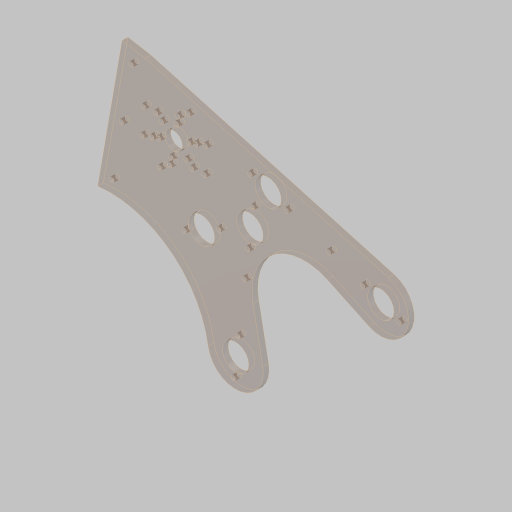
# Autodesk Inventor part: GP7-001
Saved by Autodesk Inventor 2023.5 (Build 275446000, 446)
## iProperties
Created: 2025-02-24
Part Number: GP7-001
Material: Polycarbonate, Smoke
Document SubType Name: Modeling
Designer: dlangdon
Density: 1.2 g/cm^3
Appearance: Polycarbonate - Smoked
Author: dlangdon
Autodesk Inventor part; units mm, degrees
ref_plane "YZ Plane" through (0, 0, 0) normal (1, 0, 0) x (0, 1, 0)
ref_plane "XZ Plane" through (0, 0, 0) normal (0, 1, 0) x (-1, 0, 0)
ref_plane "XY Plane" through (0, 0, 0) normal (0, 0, 1) x (1, 0, 0)
sketch "Sketch1" plane through (0, 0, 0) normal (0, 0, 1) x (1, 0, 0)
  circle A0 centre (78.7027, 64.253) radius 50.8 construction
  circle A1 centre (-78.7027, -64.253) radius 50.8 construction
  circle A2 centre (0, 0) radius 50.8 construction
  line L0 (-39.3513, -32.1265) -> (39.3513, 32.1265) construction
  line L1 (78.7027, 64.253) -> (-78.7027, -64.253) construction
  line L2 (-3.7208, 6.6498) -> (-3.7208, 50.6636) construction
  line L3 (-410.4212, -115.053) -> (454.9708, -115.053) construction
  circle A3 centre (140.9799, -57.903) radius 57.15 construction
  circle A4 centre (78.7027, 64.253) radius 14.2621
  circle A5 centre (-78.7027, -64.253) radius 14.2621
  circle A6 centre (-3.7208, 6.6498) radius 57.15 construction
  circle A7 centre (-78.7027, -64.253) radius 30.1371 construction
  circle A8 centre (78.7027, 64.253) radius 30.1371 construction
  circle A9 centre (-43.5314, 108.1291) radius 14.2621
  line L4 (-43.5314, 108.1291) -> (78.7027, 64.253) construction
  circle A10 centre (78.7027, 64.253) radius 14.2875 construction
  circle A11 centre (-78.7027, -64.253) radius 14.2875 construction
  circle A12 centre (-63.1248, 64.6795) radius 14.2621
  line L5 (-78.7027, -64.253) -> (-63.1248, 64.6795) construction
  circle A13 centre (-63.1248, 64.6795) radius 23.8316 construction
  circle A14 centre (-43.5314, 108.1291) radius 23.8316 construction
  line L6 (20.6869, 58.3256) -> (65.8317, 37.0027)
  line L7 (-49.1354, -58.4201) -> (-59.7901, -4.4114)
  arc A15 (20.6869, 58.3256) -> (-59.7901, -4.4114) centre (-3.7208, 6.6498) ccw
  line L8 (-201.842, 171.7522) -> (-176.8279, 167.3416)
  line L9 (-176.8279, 167.3416) -> (-203.2918, 17.2569) construction
  line L10 (-203.2918, 17.2569) -> (-228.306, 21.6675) construction
  line L11 (-228.306, 21.6675) -> (-201.842, 171.7522) construction
  line L12 (-247.3095, -86.1068) -> (28.2095, -134.6882) construction
  line L13 (-202.9446, 165.4987) -> (190.461, 96.1307) construction
  line L14 (-202.9446, 165.4987) -> (-247.3095, -86.1068) construction
  circle A16 centre (-145.8493, 105.3365) radius 31.75 construction
  line L15 (-65.9834, 41.02) -> (-72.6092, -13.8198) construction
  circle A17 centre (21.9247, 84.6336) radius 9.525 construction
  line L16 (-189.3349, 169.5469) -> (-215.7989, 19.4622) construction
  line L17 (-192.0916, 153.9131) -> (-213.0422, 35.096) construction
  circle A18 centre (-145.8493, 105.3365) radius 17.4625 construction
  circle A19 centre (-145.8493, 105.3365) radius 9.525
  circle A20 centre (-43.5314, 108.1291) radius 30.1816 construction
  line L18 (-201.842, 171.7522) -> (-228.306, 21.6675)
  arc A21 (65.8317, 37.0027) -> (86.8534, 93.267) centre (78.7027, 64.253) ccw
  arc A22 (-108.4816, -68.8852) -> (-49.1354, -58.4201) centre (-78.7027, -64.253) ccw
  line L19 (-145.8493, 105.3365) -> (-129.4399, 111.3091) construction
  line L20 (-111.5388, 117.8245) -> (-180.1598, 92.8485) construction
  circle A23 centre (-180.1598, 92.8485) radius 4.7625 construction
  line L21 (0, 0) -> (-3.7208, 6.6498) construction
  circle A24 centre (78.7027, 64.253) radius 28.6512 construction
  line L22 (66.0948, 38.525) -> (-49.8074, 95.3221) construction
  line L23 (85.335, 92.126) -> (-40.2299, 122.0038) construction
  line L24 (-176.8279, 167.3416) -> (86.8534, 93.267)
  line L25 (-145.8493, 105.3365) -> (-115.7736, 36.5549) construction
  circle A25 centre (-115.7736, 36.5549) radius 31.75 construction
  circle A26 centre (-115.7736, 36.5549) radius 14.2621
  line L26 (-63.1248, 64.6795) -> (-115.7736, 36.5549) construction
  circle A27 centre (-145.8493, 105.3365) radius 25.4 construction
  arc A28 (-108.4816, -68.8852) -> (-228.306, 21.6675) centre (-215.1488, -85.4777) ccw
  circle A29 centre (-145.8493, 105.3365) radius 36.5125 construction
  line L27 (-178.9408, 120.7674) -> (-145.8493, 105.3365) construction
  point P0 (-69.2963, 13.6001)
  point P1 (-202.5669, 94.5046)
  point P2 (-202.5669, 94.5046)
  point P3 (-142.817, 122.5337)
  point P4 (-159.2263, 116.5612)
  point P5 (-162.2587, 99.364)
  point P6 (-148.8816, 88.1393)
  point P7 (-132.4722, 94.1119)
  point P8 (-121.9811, 114.0238)
  point P9 (-141.4386, 130.3506)
  point P10 (-165.3068, 121.6633)
  point P11 (-169.7175, 96.6492)
  point P12 (-150.2599, 80.3224)
  point P13 (-126.3918, 89.0097)
  point P14 (-158.3373, 139.6471)
  point P15 (-180.1598, 92.8485)
  point P16 (-133.3613, 71.026)
  point P17 (-130.4184, 138.4281)
  point P18 (-161.2801, 72.245)
  point P19 (-112.7577, 89.9057)
  dimension "d7" = 101.6
  dimension "d18" = 47.6631
  dimension "d34" = 34.925
  dimension "d65" = 50.8
  dimension "d3" = 50.772
  dimension "d4" = 0
  dimension "d8" = 101.6
  dimension "d9" = 28.5242
  dimension "d10" = 101.6
  dimension "d11" = 114.3
  dimension "d12" = 114.3
  dimension "d13" = 15.875
  dimension "d14" = 15.875
  dimension "d15" = 129.8702
  dimension "d16" = 28.575
  dimension "d17" = 129.8702
  dimension "d19" = 47.6631
  dimension "d22" = 25.4
  dimension "d23" = 152.4
  dimension "d26" = 255.4869
  dimension "d27" = 63.5
  dimension "d30" = 203.2
  dimension "d31" = 10
  dimension "d32" = 19.05
  dimension "d33" = 120.65
  dimension "d35" = 19.05
  dimension "d36" = 6.35
  dimension "d40" = 360
  dimension "d44" = 9.525
  dimension "d55" = 80
  dimension "d56" = 7.62
  dimension "d58" = 57.3024
  dimension "d59" = 63.5
  dimension "d60" = 75.0697
  dimension "d61" = 59.69
  dimension "d62" = 55
  dimension "d68" = 360
  dimension "d70" = 41.275
  dimension "d71" = 60
  dimension "d82" = 360
  dimension "d87" = 360
  dimension "d89" = 45
  dimension "d90" = 6.35
  dimension "d91" = 20.955
  dimension "d92" = 107.95
  constraints: 56 end point, 26 centre point, 24 coincident, 23 point on circle, 14 tangent, 7 midpoint, 6 equal radius, 5 point on line, 4 collinear, 4 parallel, 2 horizontal, 1 concentric, 1 perpendicular, 1 vertical, 39 other
  measures "d3" angle of L2 L0
  measures "d4" distance between parallel lines of L0 L1
  measures "d8" diameter of A2
  measures "d9" diameter of A4
  measures "d10" diameter of A0
  measures "d11" diameter of A3
  measures "d12" diameter of A6
  measures "d13" radial gap between concentric circles of A5 A7
  measures "d14" radial gap between concentric circles of A4 A8
  measures "d15" distance of L4.start L4.end
  measures "d16" diameter of A10
  measures "d17" distance of L5.start L5.end
  measures "d19" diameter of A14
  measures "d22" distance of L9.end L10.end
  measures "d23" distance of L10.end L8.start
  measures "d26" distance of L13.start L12.start
  measures "d27" diameter of A16
  measures "d30" distance from line of point (0, 0) L9
  measures "d31" angle of L3 L12
  measures "d32" diameter of A17
  measures "d33" distance of L17.start L17.end
  measures "d35" diameter of A19
  measures "d36" radial gap between concentric circles of A14 A20
  measures "d44" diameter of A23
  measures "d55" angle of L1 L21
  measures "d56" distance of L21.start L21.end
  measures "d58" diameter of A24
  measures "d59" diameter of A25
  measures "d60" distance of L19.start L25.end
  measures "d61" distance of L26.start L26.end
  measures "d62" angle of L15 L26
  measures "d70" distance from line of L9 L19.start
  measures "d71" angle of L9 L20
  measures "d89" angle of L20 L27
  measures "d90" distance between parallel lines of L8 L13
  measures "d91" distance from line of L24 L4.start
  measures "d92" radius of A28
extrude "Extrusion1" add sketch "Sketch1" along normal blind 6.35
hole "Hole1" at (21.9247, 84.6336, 0) at (-192.0916, 153.9131, 0) at (-202.5669, 94.5046, 0) at (-213.0422, 35.096, 0) at (-129.4399, 111.3091, 0) at (-142.817, 122.5337, 0) at (-159.2263, 116.5612, 0) at (-162.2587, 99.364, 0) at (-148.8816, 88.1393, 0) at (-132.4722, 94.1119, 0) at (-111.5388, 117.8245, 0) at (-180.1598, 92.8485, 0) at (-150.2599, 80.3224, 0) at (-169.7175, 96.6492, 0) at (-165.3068, 121.6633, 0) at (-141.4386, 130.3506, 0) at (-121.9811, 114.0238, 0) at (-126.3918, 89.0097, 0) at (-69.2963, 13.6001, 0) at (-178.9408, 120.7674, 0) at (-130.4184, 138.4281, 0) at (-112.7577, 89.9057, 0) at (-161.2801, 72.245, 0) direction (0, 0, 1) diameter 5.1054 end through all clearance for "Flat Head Machine Screw (82)" size "#10" standard "Ansi Unified Screw Threads"
sketch "Sketch2" plane through (0, 0, 6.35) normal (0, 0, 1) x (1, 0, 0)
  circle A0 centre (-126.3918, 89.0097) radius 2.5527 construction
  circle A1 centre (-141.4386, 130.3506) radius 2.5527 construction
  circle A2 centre (-169.7175, 96.6492) radius 2.5527 construction
  circle A3 centre (-180.1598, 92.8485) radius 2.5527 construction
  circle A4 centre (-132.4722, 94.1119) radius 2.5527 construction
  circle A5 centre (-162.2587, 99.364) radius 2.5527 construction
  circle A6 centre (-142.817, 122.5337) radius 2.5527 construction
  circle A7 centre (-213.0422, 35.096) radius 2.5527 construction
  circle A8 centre (-192.0916, 153.9131) radius 2.5527 construction
  circle A9 centre (21.9247, 84.6336) radius 2.5527 construction
  circle A10 centre (-202.5669, 94.5046) radius 2.5527 construction
  circle A11 centre (-129.4399, 111.3091) radius 2.5527 construction
  circle A12 centre (-159.2263, 116.5612) radius 2.5527 construction
  circle A13 centre (-148.8816, 88.1393) radius 2.5527 construction
  circle A14 centre (-111.5388, 117.8245) radius 2.5527 construction
  circle A15 centre (-150.2599, 80.3224) radius 2.5527 construction
  circle A16 centre (-165.3068, 121.6633) radius 2.5527 construction
  circle A17 centre (-121.9811, 114.0238) radius 2.5527 construction
  circle A18 centre (-69.2963, 13.6001) radius 2.5527 construction
  line L0 (-49.1354, -58.4201) -> (-59.7901, -4.4114) construction
  arc A19 (20.6869, 58.3256) -> (-59.7901, -4.4114) centre (-3.7208, 6.6498) ccw construction
  line L1 (20.6869, 58.3256) -> (65.8317, 37.0027) construction
  arc A20 (65.8317, 37.0027) -> (86.8534, 93.267) centre (78.7027, 64.253) ccw construction
  line L2 (86.8534, 93.267) -> (-176.8279, 167.3416) construction
  line L3 (-176.8279, 167.3416) -> (-201.842, 171.7522) construction
  line L4 (-201.842, 171.7522) -> (-228.306, 21.6675) construction
  arc A21 (-108.4816, -68.8852) -> (-228.306, 21.6675) centre (-215.1488, -85.4777) ccw construction
  arc A22 (-108.4816, -68.8852) -> (-49.1354, -58.4201) centre (-78.7027, -64.253) ccw construction
  circle A23 centre (-63.1248, 64.6795) radius 14.2621 construction
  circle A24 centre (-145.8493, 105.3365) radius 9.525 construction
  circle A25 centre (-115.7736, 36.5549) radius 14.2621 construction
  circle A26 centre (-43.5314, 108.1291) radius 14.2621 construction
  circle A27 centre (-78.7027, -64.253) radius 14.2621 construction
  circle A28 centre (78.7027, 64.253) radius 14.2621 construction
  line L5 (-76.1815, -43.3863) -> (-81.2238, -85.1198) construction
  line L6 (-134.3127, 26.6514) -> (-97.2345, 46.4583) construction
  line L7 (-60.6036, 85.5463) -> (-65.6459, 43.8128) construction
  line L8 (-63.314, 115.2301) -> (-23.7487, 101.0281) construction
  line L9 (58.92, 71.354) -> (98.4853, 57.152) construction
  circle A29 centre (-63.1248, 64.6795) radius 14.2621 construction
  line L10 (-43.5314, 108.1291) -> (-63.1248, 64.6795) construction
  line L11 (-43.5314, 108.1291) -> (78.7027, 64.253) construction
  line L12 (-63.1248, 64.6795) -> (-115.7736, 36.5549) construction
  line L13 (-63.1248, 64.6795) -> (-78.7027, -64.253) construction
  circle A30 centre (-112.7577, 89.9057) radius 2.5527 projected
  point P0 (0, 0)
  point P1 (-116.0598, 70.5176)
  point P2 (-113.1961, 73.3575)
  dimension "d72" = 42.037
  constraints: 19 end point, 14 coincident, 5 collinear, 5 midpoint, 4 equal length, 1 other
  measures "d72" distance of L5.start L5.end
hole "Hole2" at (-76.1815, -43.3863, 6.35) at (-97.2345, 46.4583, 6.35) at (-81.2238, -85.1198, 6.35) at (-134.3127, 26.6514, 6.35) at (-65.6459, 43.8128, 6.35) at (-60.6036, 85.5463, 6.35) at (-23.7487, 101.0281, 6.35) at (-63.314, 115.2301, 6.35) at (98.4853, 57.152, 6.35) at (58.92, 71.354, 6.35) direction (0, 0, -1) diameter 5.1054 end through all clearance for "Flat Head Machine Screw (82)" size "#10" standard "Ansi Unified Screw Threads"
body "Solid1"
